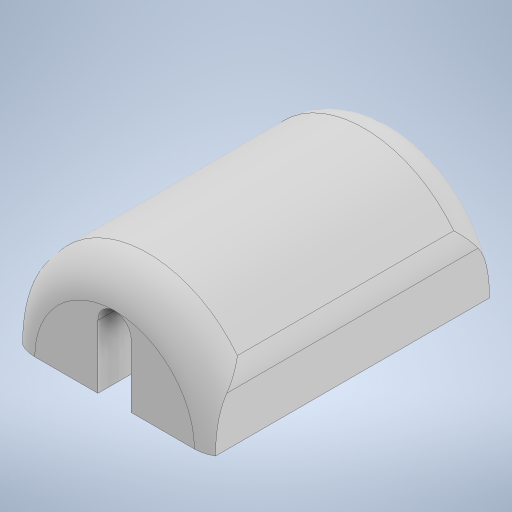
# Autodesk Inventor part: OptoPair
Saved by Autodesk Inventor 2024 (Build 280153000, 153)
## iProperties
Created: 2025-10-06
Part Number: OptoPair
Material: Типовые
Document SubType Name: Modeling
Designer: fm
Density: 1 g/cm^3
Appearance: По умолчанию
Author: fm
Autodesk Inventor part; units mm, degrees
ref_plane "YZ Plane" through (0, 0, 0) normal (1, 0, 0) x (0, 1, 0)
ref_plane "XZ Plane" through (0, 0, 0) normal (0, 1, 0) x (-1, 0, 0)
ref_plane "XY Plane" through (0, 0, 0) normal (0, 0, 1) x (1, 0, 0)
sketch "Эскиз1" plane through (0, 0, 0) normal (0, 0, 1) x (1, 0, 0)
  arc A0 (2.3, 1.5969) -> (-2.3, 1.5969) centre (0, 0) ccw
  line L0 (-2.3, 0) -> (2.3, 0) construction
  line L1 (-2.3, 1.5969) -> (-2.3, -1.5969)
  line L2 (2.3, 1.5969) -> (2.3, -1.5969)
  arc A1 (-2.3, -1.5969) -> (2.3, -1.5969) centre (0, 0) ccw
  line L3 (0, 1.9) -> (0, -1.9) construction
  circle A2 centre (0, 1.9) radius 0.5
  circle A3 centre (0, -1.9) radius 0.5
  line L4 (-0.5, 1.9) -> (-0.5, -1.9)
  line L5 (0.5, 1.9) -> (0.5, -1.9)
  line L6 (-2.9, 1.7748) -> (-2.9, -1.7748)
  arc A4 (-2.9, -1.7748) -> (2.9, -1.7748) centre (0, 0) ccw
  line L7 (2.9, -1.7748) -> (2.9, 1.7748)
  arc A5 (2.9, 1.7748) -> (-2.9, 1.7748) centre (0, 0) ccw
  line L8 (-2.9, 0) -> (2.9, 0)
  point P0 (0, 0)
  point P1 (-0.5, 0)
  point P2 (0.5, 0)
  point P3 (2.3, 0)
  point P4 (-2.3, 0)
  dimension "d1" = 4.6
  dimension "d2" = 2.8
  dimension "d3" = 3.8
  dimension "d4" = 1
  dimension "d5" = 1
  dimension "d6" = 0.6
  dimension "d7" = 3.4
  constraints: 18 end point, 13 point on circle, 6 centre point, 6 midpoint, 5 coincident, 5 vertical, 2 horizontal, 2 tangent, 3 other
  measures "d1" distance of L0.end L0.start
  measures "d2" radius of A0
  measures "d3" distance of L3.start L3.end
  measures "d4" diameter of A2
  measures "d5" diameter of A3
  measures "d6" radial gap between concentric circles of A0 A5
  measures "d7" radius of A5
extrude "Выдавливание1" add sketch "Эскиз1" against normal blind 1 contours L2 L8 L5 A2 L4 L1 A0 | A0 L1 L8 L6 A5 L7 L2
extrude "Выдавливание2" add sketch "Эскиз1" against normal blind 2.2 from surface at -1 contours A0 L1 L8 L6 A5 L7 L2
sketch "Эскиз2" plane through (0, 0, -3.2) normal (0, 0, -1) x (-1, 0, 0)
  line L0 (-2.9, 0) -> (-2.3, 0) projected
  line L1 (-2.3, 0) -> (-2.3, 1.5969) projected
  arc A0 (2.3, 1.5969) -> (-2.3, 1.5969) centre (0, 0) ccw projected
  line L2 (2.3, 1.5969) -> (2.3, 0) projected
  line L3 (2.3, 0) -> (2.9, 0) projected
  line L4 (2.9, 0) -> (2.9, 1.7748) projected
  arc A1 (2.9, 1.7748) -> (-2.9, 1.7748) centre (0, 0) ccw projected
  line L5 (-2.9, 1.7748) -> (-2.9, 0) projected
  circle A2 centre (0, 0) radius 1.8
  circle A3 centre (0, 0) radius 2.2
  line L6 (-2.9, 0) -> (2.9, 0)
  line L7 (0, -1.3) -> (0, 1.3) construction
  circle A4 centre (0, 1.3) radius 0.5
  line L8 (0.5, 0) -> (0.5, 1.3)
  line L9 (-0.5, 0) -> (-0.5, 1.3)
  point P0 (0, 0)
  point P1 (2.3, 0)
  point P2 (-2.3, 0)
  point P3 (-1.8, 0)
  point P4 (0, 1.8)
  point P5 (0.2522, 1.7317)
  point P6 (1.8, 0)
  point P7 (-2.2, 0)
  point P8 (2.2, 0)
  point P9 (-2.3, 0)
  point P10 (2.3, 0)
  dimension "d12" = 3.6
  dimension "d13" = 4.4
  dimension "d14" = 2.6
  dimension "d15" = 1
  constraints: 8 end point, 3 centre point, 3 coincident, 2 midpoint, 2 point on circle, 2 point on line, 2 tangent, 2 vertical, 1 collinear, 1 perpendicular
  measures "d12" diameter of A2
  measures "d13" diameter of A3
  measures "d14" distance of L7.start L7.end
  measures "d15" diameter of A4
extrude "Выдавливание3" add sketch "Эскиз2" along normal blind 3.3 contours L5 A1 L4 L3 L2 A0 L1 L0 | L1 A0 L2 L6 A3 | A3 L6 A2 picked at (-2.0303, 0.309)
extrude "Выдавливание4" add sketch "Эскиз2" along normal blind 1 from surface at 3.3 contours L5 A1 L4 L3 L2 A0 L1 L0 | L1 A0 L2 L6 A3
extrude "Выдавливание5" add sketch "Эскиз2" along normal blind 1 from surface at 4.3 contours L5 A1 L4 L3 L2 A0 L1 L0 | L1 A0 L2 L6 A3 | A3 L6 A2 | A2 A4 L9 L6 | L6 L8 A4 A2 picked at (-2.0303, 0.309)
fillet "Сопряжение1" radius 1 4 edges at (0, 3.4, 0) (0, 3.4, -8.5) (2.9, 1.7748, -4.25) (-2.9, 1.7748, -4.25)
